Hole Hook  Small (Autodesk Fusion 360 design; units mm, degrees)
Autodesk Fusion 360 part; units mm, degrees
sketch "Sketch1" plane through (0, 0, 0) normal (0, 1, 0) x (1, 0, 0)
  circle A0 centre (0, 0) radius 7.2
  circle A1 centre (0, 0) radius 2.55
  line L0 (7.2, -0.0062) -> (2.55, -0.0062)
  line L1 (2.55, -0.0062) -> (2.55, -28.2062)
  line L2 (2.55, -28.2062) -> (7.2, -28.2062)
  line L3 (7.2, -28.2062) -> (7.2, -0.0062)
  line L4 (7.2, -28.2062) -> (-3.3, -28.2062)
  line L5 (-3.3, -28.2062) -> (-3.3, -23.5562)
  line L6 (-3.3, -23.5562) -> (7.2, -23.5562)
  line L7 (7.2, -23.5562) -> (7.2, -28.2062)
  line L8 (2.55, -0.0062) -> (-7.2, -0.0062)
  line L9 (7.2, -5.8) -> (7.2, -1.15)
  line L10 (7.2, -23.5562) -> (12.2, -23.5562)
  line L11 (12.2, -23.5562) -> (12.2, -28.2062)
  line L12 (12.2, -28.2062) -> (7.2, -28.2062)
  line L13 (7.2, -28.2062) -> (7.2, -23.5562)
  line L14 (7, -3.5562) -> (12.2, -3.5562)
  line L15 (12.2, -3.5562) -> (12.2, 1.0938)
  line L16 (12.2, 1.0938) -> (7, 1.0938)
  line L17 (7, 1.0938) -> (7, -3.5562)
  dimension "d1" = 14.4
  dimension "d2" = 5.1
  dimension "d3" = 4.65
  dimension "d4" = 28.2
  dimension "d5" = 10.5
  dimension "d21" = 5
  dimension "d37" = 5.2
  dimension "d38" = 4.65
  dimension "d39" = 20
  constraint coincident A0.centre A1.centre
  constraint concentric A0 A1
  constraint horizontal L0
  constraint vertical L1
  constraint horizontal L2
  constraint vertical L3
  constraint coincident A0 L0.start
  constraint coincident A1 L0.end
  constraint horizontal L4
  constraint vertical L5
  constraint horizontal L6
  constraint vertical L7
  constraint coincident A0 L8.end
  constraint perpendicular L1 L8
  constraint vertical L9
  constraint coincident L3 L9.end
  constraint horizontal L10
  constraint vertical L11
  constraint horizontal L12
  constraint vertical L13
  constraint horizontal L14
  constraint vertical L15
  constraint horizontal L16
  constraint vertical L17
  constraint collinear L11 L15
  measures "d1" diameter of A0
  measures "d2" diameter of A1
  measures "d3" horizontal distance of L1.end L2.end
  measures "d4" vertical distance of L0.start L2.end
  measures "d5" distance of L2.end L4.end
  measures "d21" distance of L6.end L10.end
  measures "d37" distance of L14.start L14.end
  measures "d38" distance of L14.start L16.end
  measures "d39" distance of L10 L14
extrude "Extrude1" add sketch "Sketch1" along normal blind 4.65 contours A0 L0 L16 L17 | A0 L3 L9 L14 L17 | A0 L0 L17 | A0 L3 L9 L14 L15 L16 | A0 L1 L3 L6 L9 L14 L17 | A0 L0 L1 L17 | A0 A1 L0 L8 L16 L17 | L1 L2 L3 L4 L6 L7 L13 | L1 L4 L5 L6 | L3 L7 L10 L11 L12 L13 makes body 1
fillet "Fillet3" radius 2 2 edges at (-0.375, 4.65, 23.5562) (-0.375, 0, 23.5562) on bodies 1
sketch "Sketch2" plane through (0, 0, 0) normal (0, 1, 0) x (1, 0, 0)
  line L0 (14.397, -23.55) -> (19.397, -23.55)
  line L1 (19.397, -23.55) -> (19.397, -3.55)
  line L2 (19.397, -3.55) -> (14.397, -3.55)
  line L3 (14.397, -3.55) -> (14.397, -23.55)
  line L4 (14.397, -3.55) -> (49.397, -3.55)
  line L5 (49.397, -3.55) -> (49.397, -6.55)
  line L6 (49.397, -6.55) -> (14.397, -6.55)
  line L7 (14.397, -6.55) -> (14.397, -3.55)
  dimension "d22" = 5
  dimension "d23" = 20
  dimension "d24" = 35
  dimension "d25" = 3
  constraint horizontal L0
  constraint vertical L1
  constraint horizontal L2
  constraint vertical L3
  constraint horizontal L4
  constraint vertical L5
  constraint horizontal L6
  constraint vertical L7
  measures "d22" distance of L0.start L0.end
  measures "d23" distance of L0.start L2.end
  measures "d24" distance of L2.end L4.end
  measures "d25" distance of L2.end L6.end
extrude "Extrude2" add sketch "Sketch2" along normal blind 35 separate body contours L1 L2 L3 L4 L6 L7 | L1 L4 L5 L6 makes body 2
extrude "Extrude3" add sketch "Sketch2" along normal blind 35 contours L0 L1 L3 L6 bodies 2
sketch "Sketch3" plane through (0, 0, 0) normal (0, 0, 1) x (1, 0, 0)
  circle A0 centre (34.5231, 17.5) radius 6
  dimension "d31" = 12
  measures "d31" diameter of A0
extrude "Extrude4" cut sketch "Sketch3" along normal blind 13 bodies 2
chamfer "Chamfer1" distance 15 angle 45 2 edges at (16.897, 35, 23.55) (16.897, 0, 23.55) on bodies 2
fillet "Fillet5" radius 8.5 2 edges at (49.397, 0, 5.05) (49.397, 35, 5.05) on bodies 2
